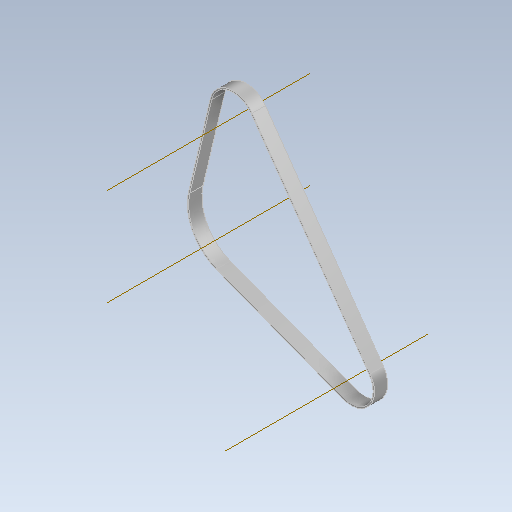
# Autodesk Inventor part: Зубчатый ремень
Saved by Autodesk Inventor 2021 (Build 250183000, 183)
## iProperties
Created: 2021-06-17
Part Number: Зубчатый ремень
Material: Rubber
Document SubType Name: Modeling
Designer: panda
Density: 1 g/cm^3
Appearance: Rubber - Black - Version 1.1
CustomPartVersion: 1
Author: panda
Autodesk Inventor part; units mm, degrees
sketch "Эскизная траектория" plane through (0, 0, 0) normal (0, 0, 1) x (1, 0, 0)
  arc A0 (26.3905, 58.6932) -> (-31.4656, 47.4707) centre (0, 40) ccw
  arc A1 (158.3955, -230.1866) -> (196.3905, -181.3068) centre (170, -200) ccw
  arc A2 (-62.9312, -85.0587) -> (-23.209, -160.3732) centre (0, -100) ccw
  line L0 (-62.9312, -85.0587) -> (-31.4656, 47.4707)
  line L1 (26.3905, 58.6932) -> (196.3905, -181.3068)
  line L2 (158.3955, -230.1866) -> (-23.209, -160.3732)
  constraints: 6 end point, 6 point on circle, 3 centre point
ref_plane "Плоскость сечения" through (-31.4656, 47.4707, 0) normal (-0.231, -0.973, 0) x (0, 0, 1)
ref_plane "РабПлоскость2" through (0, 40, 0) normal (-1, 0, 0) x (0, 0, 1)
ref_plane "РабПлоскость3" through (170, -200, 0) normal (-0.4393, 0.8983, 0) x (0, 0, 1)
ref_plane "РабПлоскость4" through (0, -100, 0) normal (0.8859, -0.4639, 0) x (0, 0, 1)
sketch "Сечение" plane through (-31.4656, 47.4707, 0) normal (-0.231, -0.973, 0) x (0, 0, 1)
  line L0 (-9.525, 1.3462) -> (9.525, 1.3462)
  line L1 (9.525, 1.3462) -> (9.525, -0.6858)
  line L2 (9.525, -0.6858) -> (-9.525, -0.6858)
  line L3 (-9.525, -0.6858) -> (-9.525, 1.3462)
  line L4 (-9.525, 0) -> (9.525, 0) construction
  point P0 (0, 0)
  point P1 (0, 0)
  dimension "d0" = 19.05
  dimension "d4" = 0.6858
  dimension "d5" = 1.3462
  constraints: 10 end point, 2 parallel, 2 point on line, 1 coincident, 1 horizontal, 1 midpoint, 1 perpendicular, 1 other
  measures "d0" distance between parallel lines of L1 L3
  measures "d4" distance between parallel lines of L2 L4
  measures "d5" distance between parallel lines of L4 L0
sweep "Ремень" add profiles "Сечение" path "Эскизная траектория"
equation "\"d0\" = da_B"
equation "\"d4\" = da_a"
equation "\"d5\" = da_a2"
equation "\"da_B\" = 19.05"
equation "\"da_pb\" = 12.7"
equation "\"da_L\" = 874.5532"
equation "\"da_a\" = 0.6858"
equation "\"da_S\" = 6.1214"
equation "\"da_Beta\" = 20deg"
equation "\"da_Ht\" = 2.286"
equation "\"da_H\" = 4.318"
equation "\"da_a2\" = 1.3462"
body "Solid1"
